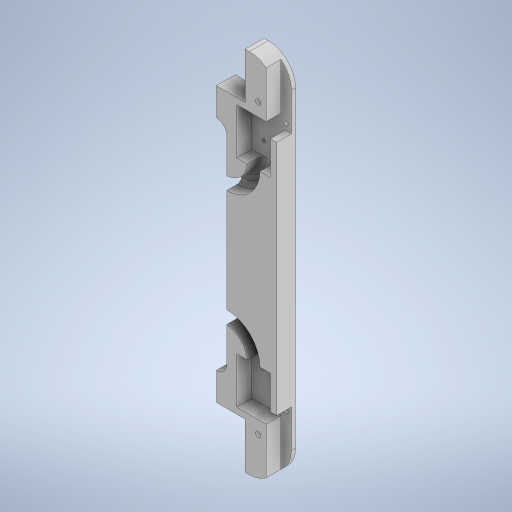
# Autodesk Inventor part: front_part
Saved by Autodesk Inventor 2023 (Build 270158000, 158)
## iProperties
Created: 2026-02-11
Part Number: front_part
Material: Типовые
Document SubType Name: Modeling
Designer: garin
Density: 1 g/cm^3
Appearance: По умолчанию
Author: garin
Autodesk Inventor part; units mm, degrees
ref_plane "YZ Plane" through (0, 0, 0) normal (1, 0, 0) x (0, 1, 0)
ref_plane "XZ Plane" through (0, 0, 0) normal (0, 1, 0) x (-1, 0, 0)
ref_plane "XY Plane" through (0, 0, 0) normal (0, 0, 1) x (1, 0, 0)
sketch "Эскиз1" plane through (0, 0, 0) normal (0, 0, 1) x (1, 0, 0)
  line L0 (117.5766, 0) -> (-136.0871, 0) construction
  line L1 (0, 117.7947) -> (0, -152.0118) construction
  line L2 (0, 0) -> (90, 0) construction
  line L3 (65.2, 57.2) -> (61.2, 57.2) construction
  line L4 (65.2, 57.2) -> (65.2, 52.2) construction
  line L5 (75, 65.5) -> (75, 87.5)
  line L6 (75, 87.5) -> (77, 87.5)
  arc A0 (90, 74.5) -> (77, 87.5) centre (77, 74.5) ccw
  line L7 (90, 74.5) -> (90, 0)
  circle A1 centre (65.2, 57.2) radius 2.1
  circle A2 centre (81.1924, 78.6924) radius 2.1
  line L8 (90, 63.5) -> (90, 65.5)
  line L9 (75, 65.5) -> (61.2, 65.5)
  line L10 (66.2, 29.1) -> (66.2, 36.5)
  line L11 (66.2, 24.1) -> (66.2, 0)
  line L12 (66.2, 29.1) -> (66.2, 24.1)
  line L13 (71, 62.5) -> (71, 45.5)
  line L14 (71, 45.5) -> (71, 56.5)
  line L15 (87, 56.5) -> (87, 45.5)
  line L16 (87, 45.5) -> (74.2, 45.5)
  line L17 (74.2, 45.5) -> (74.2, 56.5)
  line L18 (74.2, 56.5) -> (87, 56.5)
  line L19 (87, 56.5) -> (87, 45.5)
  line L20 (87, 45.5) -> (87, 40.5)
  line L21 (87, 40.5) -> (71, 40.5)
  line L22 (71, 40.5) -> (71, 45.5)
  line L23 (87, 40.5) -> (79, 40.5)
  arc A3 (66.2, 24.7) -> (82, 40.5) centre (66.2, 40.5) ccw
  arc A4 (66.2, 30.7) -> (76, 40.5) centre (65.5077, 41.1923) ccw
  line L24 (80.6, 45.5) -> (83.35, 45.5)
  line L25 (83.35, 45.5) -> (76.85, 45.5)
  line L26 (74.2, 45.5) -> (73.7, 45.5)
  circle A5 centre (76.85, 47) radius 0.8
  circle A6 centre (83.35, 47) radius 0.8
  line L27 (87, 45.5) -> (87, 55.9)
  line L28 (65.2, -57.2) -> (61.2, -57.2) construction
  line L29 (65.2, -57.2) -> (65.2, -52.2) construction
  line L30 (75, -65.5) -> (75, -87.5)
  line L31 (75, -87.5) -> (77, -87.5)
  arc A7 (77, -87.5) -> (90, -74.5) centre (77, -74.5) ccw
  line L32 (90, -74.5) -> (90, 0)
  circle A8 centre (65.2, -57.2) radius 2.1
  circle A9 centre (81.1924, -78.6924) radius 2.1
  line L33 (90, -63.5) -> (90, -65.5)
  line L34 (75, -65.5) -> (61.2, -65.5)
  line L35 (71, -62.5) -> (71, -45.5)
  line L36 (71, -45.5) -> (71, -56.5)
  line L37 (87, -56.5) -> (87, -45.5)
  line L38 (87, -45.5) -> (74.2, -45.5)
  line L39 (74.2, -45.5) -> (74.2, -56.5)
  line L40 (74.2, -56.5) -> (87, -56.5)
  line L41 (87, -56.5) -> (87, -45.5)
  line L42 (87, -45.5) -> (87, -40.5)
  line L43 (87, -40.5) -> (71, -40.5)
  line L44 (71, -40.5) -> (71, -45.5)
  line L45 (87, -40.5) -> (79, -40.5)
  arc A10 (82, -40.5) -> (66.2, -24.7) centre (66.2, -40.5) ccw
  arc A11 (76, -40.5) -> (66.2, -30.7) centre (65.5077, -41.1923) ccw
  line L46 (80.6, -45.5) -> (83.35, -45.5)
  line L47 (83.35, -45.5) -> (76.85, -45.5)
  line L48 (74.2, -45.5) -> (73.7, -45.5)
  circle A12 centre (76.85, -47) radius 0.8
  circle A13 centre (83.35, -47) radius 0.8
  line L49 (87, -45.5) -> (87, -55.9)
  line L50 (87, -56.5) -> (90, -56.5)
  circle A14 centre (87.508, -59.5) radius 1
  circle A15 centre (81.1924, 68.6924) radius 1.3
  circle A16 centre (81.1924, -68.6924) radius 1.3
  line L51 (61.2, 65.5) -> (61.2, 52.2)
  arc A17 (66.2, 47.2) -> (61.2, 52.2) centre (61.2, 47.2) ccw
  line L52 (66.2, 47.2) -> (66.2, 36.5)
  line L53 (66.2, -29.1) -> (66.2, -36.5)
  line L54 (66.2, -24.1) -> (66.2, 0)
  line L55 (66.2, -29.1) -> (66.2, -24.1)
  line L56 (61.2, -65.5) -> (61.2, -52.2)
  arc A18 (61.2, -52.2) -> (66.2, -47.2) centre (61.2, -47.2) ccw
  line L57 (66.2, -47.2) -> (66.2, -36.5)
  line L58 (85, -68.6924) -> (85, -84.747)
  line L59 (71, -62.5) -> (85, -62.5)
  line L60 (85, -62.5) -> (85, -68.6924)
  circle A19 centre (87.508, 59.5) radius 1
  line L61 (85, 68.6924) -> (85, 84.747)
  line L62 (71, 62.5) -> (85, 62.5)
  line L63 (85, 62.5) -> (85, 68.6924)
  line L64 (87, 56.5) -> (90, 56.5)
  point P0 (60.2, 65.5)
  point P1 (74.2, 55.9)
  point P2 (87, 82.8066)
  point P3 (60.2, -65.5)
  point P4 (74.2, -55.9)
  point P5 (87, -82.8066)
  point P6 (81.1924, 67.6924)
  point P7 (81.1924, -67.6924)
  point P8 (87.75, -59.5)
  dimension "d6" = 90
  dimension "d11" = 4
  dimension "d12" = 5
  dimension "d14" = 13
  dimension "d20" = 4.2
  dimension "d64" = 7.4
  dimension "d76" = 16
  dimension "d77" = 17
  dimension "d78" = 11
  dimension "d79" = 12.8
  dimension "d80" = 5
  dimension "d81" = 8
  dimension "d88" = 0.5
  dimension "d92" = 10.4
  dimension "d105" = 2.6
  constraints: 130 end point, 55 symmetric about line, 20 centre point, 19 point on circle, 17 point on line, 7 horizontal, 6 perpendicular, 5 coincident, 5 vertical, 3 midpoint, 3 parallel, 2 collinear, 1 tangent, 9 other
  measures "d6" distance of L2.start L2.end
  measures "d11" distance of L3.start L3.end
  measures "d12" distance of L3.start L4.end
  measures "d14" radius of A0
  measures "d20" diameter of A1
  measures "d64" distance of L10.start L10.end
  measures "d76" distance of L15.end L13.end
  measures "d77" distance of L13.end L13.start
  measures "d78" distance of L14.start L14.end
  measures "d79" distance of L17.end L18.end
  measures "d80" distance of L15.end L20.end
  measures "d81" distance of L20.end L23.end
  measures "d88" distance of L16.end L26.end
  measures "d92" distance of L15.end L27.end
  measures "d105" diameter of A15
extrude "Выдавливание13" add sketch "Эскиз1" along normal blind 9 contours L5 L6 A0 L61 L63 L62 L13 L22 L21 A4 L10 L52 A17 L51 L9 | L7 L32 L50 L37 L42 L43 A10 L55 L54 L11 L12 A3 L21 L20 L15 L64 | A7 L31 L30 L34 L56 A18 L57 L53 A11 L43 L44 L35 L59 L60 L58 | A1 | A2 | A8 | A9
extrude "Выдавливание16" add sketch "Эскиз1" along normal blind 2 contours A0 L7 L64 L18 L17 L16 L20 L21 L22 L13 L62 L63 L61 | A4 L21 A3 L12 L10 | L15 L16 L17 L18 | L32 A7 L58 L60 L59 L35 L44 L43 L42 L38 L39 L40 L50 | L40 L39 L38 L37 | A10 L43 A11 L53 L55
fillet "Сопряжение3" radius 2 4 edges at (72.943, -33.757, 2) (77.3723, -29.3277, 2) (77.3723, 29.3277, 2) (72.943, 33.757, 2)
